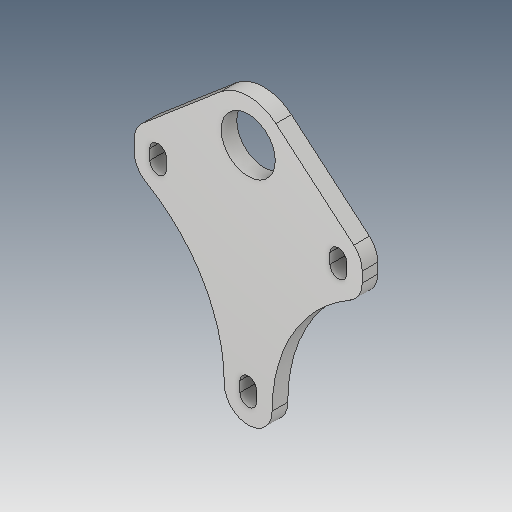
# Autodesk Inventor part: POTplate
Saved by Autodesk Inventor 2019.4 (Build 234330000, 330)
## iProperties
Created: 2019-06-16
Part Number: POTplate
Material: アルミニウム 2014-T4
Document SubType Name: Modeling
Designer: AzLIer
Density: 2.8 g/cm^3
Appearance: サテン
Mass: 11.1022 g
Surface Area: 33.0768 cm^2
Volume: 3.96506 cm^3
Author: AzLIer
Autodesk Inventor part; units mm, degrees
ref_plane "YZ Plane" through (0, 0, 0) normal (1, 0, 0) x (0, 1, 0)
ref_plane "XZ Plane" through (0, 0, 0) normal (0, 1, 0) x (-1, 0, 0)
ref_plane "XY Plane" through (0, 0, 0) normal (0, 0, 1) x (1, 0, 0)
sketch "スケッチ1" plane through (0, 0, 0) normal (0, 0, 1) x (1, 0, 0)
  circle A0 centre (0, 0) radius 5.2
  line L0 (25, -50) -> (-25, -50)
  line L1 (-25, -50) -> (-25, 50)
  line L2 (-25, 50) -> (25, 50)
  line L3 (25, 50) -> (25, -50)
  line L4 (25, -50) -> (-25, 50) construction
  line L5 (-25, -50) -> (25, 50) construction
  dimension "d0" = 10.4
  dimension "d1" = 50
  dimension "d2" = 100
  constraints: 12 end point, 2 midpoint, 2 parallel, 1 centre point, 1 coincident, 1 horizontal, 1 perpendicular
  measures "d0" diameter of A0
  measures "d1" distance of L1.end L2.end
  measures "d2" distance of L0.end L1.end
extrude "押し出し1" add sketch "スケッチ1" along normal blind 3
sketch "スケッチ2" plane through (0, 0, 3) normal (0, 0, 1) x (1, 0, 0)
  circle A0 centre (17.3198, -9.9987) radius 1.25 construction
  circle A1 centre (-17.3213, -10.0013) radius 1.25 construction
  circle A2 centre (0.0015, -40) radius 1.25 construction
  line L0 (-17.3213, -10.0013) -> (-17.3213, -12.0013) construction
  line L1 (-18.9213, -10.0013) -> (-18.9213, -12.0013)
  line L2 (-15.7213, -12.0013) -> (-15.7213, -10.0013)
  arc A3 (-15.7213, -10.0013) -> (-18.9213, -10.0013) centre (-17.3213, -10.0013) ccw
  arc A4 (-18.9213, -12.0013) -> (-15.7213, -12.0013) centre (-17.3213, -12.0013) ccw
  line L3 (0.0015, -40) -> (0.0015, -42) construction
  line L4 (-1.5985, -40) -> (-1.5985, -42)
  line L5 (1.6015, -42) -> (1.6015, -40)
  arc A5 (1.6015, -40) -> (-1.5985, -40) centre (0.0015, -40) ccw
  arc A6 (-1.5985, -42) -> (1.6015, -42) centre (0.0015, -42) ccw
  line L6 (17.3198, -9.9987) -> (17.3198, -11.9987) construction
  line L7 (15.7198, -9.9987) -> (15.7198, -11.9987)
  line L8 (18.9198, -11.9987) -> (18.9198, -9.9987)
  arc A7 (18.9198, -9.9987) -> (15.7198, -9.9987) centre (17.3198, -9.9987) ccw
  arc A8 (15.7198, -11.9987) -> (18.9198, -11.9987) centre (17.3198, -11.9987) ccw
  circle A9 centre (0, 0) radius 5.2 projected
  arc A10 (5.3111, 6.2476) -> (-5.3114, 6.2473) centre (0, 0) ccw
  line L9 (-12.7213, -12.0013) -> (-12.7213, -10.0013)
  arc A11 (-20.3008, -6.4967) -> (-21.9213, -10.0013) centre (-17.3213, -10.0013) ccw
  line L10 (-21.9213, -10.0013) -> (-21.9213, -12.0013)
  arc A12 (-21.9213, -12.0013) -> (-21.3048, -14.3016) centre (-17.3213, -12.0013) ccw
  line L11 (21.9198, -11.9987) -> (21.9198, -9.9987)
  arc A13 (21.9198, -9.9987) -> (20.2992, -6.494) centre (17.3198, -9.9987) ccw
  line L12 (12.7198, -9.9987) -> (12.7198, -11.9987)
  arc A14 (21.3037, -14.2984) -> (21.9198, -11.9987) centre (17.3198, -11.9987) ccw
  line L13 (4.6015, -40) -> (4.6015, -42)
  arc A15 (-3.9821, -44.3003) -> (3.9854, -44.2997) centre (0.0015, -42) ccw
  line L14 (-4.5985, -42) -> (-4.5985, -40)
  arc A16 (4.6015, -40) -> (-4.5985, -40) centre (0.0015, -40) ccw
  line L15 (-20.3008, -6.4967) -> (-5.3114, 6.2473)
  line L16 (5.3111, 6.2476) -> (20.2992, -6.494)
  line L17 (21.3037, -14.2984) -> (3.9854, -44.2997)
  line L18 (-3.9821, -44.3003) -> (-21.3048, -14.3016)
  point P0 (-17.3213, -11.0013)
  point P1 (0.0015, -41)
  point P2 (17.3198, -10.9987)
  dimension "d5" = 1.6
  dimension "d6" = 2
  dimension "d7" = 3
  dimension "d8" = 3
  dimension "d9" = 3
  dimension "d10" = 3
  constraints: 44 end point, 26 point on circle, 20 tangent, 13 centre point, 10 parallel, 3 midpoint, 2 equal radius, 1 vertical, 1 other
  measures "d5" radius of A4
  measures "d6" distance of L3.start L3.end
  measures "d7" radial gap between concentric circles of A9 A10
  measures "d8" radial gap between concentric circles of A4 A12
  measures "d9" radial gap between concentric circles of A8 A14
  measures "d10" distance between parallel lines of L5 L13
extrude "押し出し2" cut sketch "スケッチ2" against normal blind 3 keep common part
sketch "スケッチ3" plane through (0, 0, 3) normal (0, 0, 1) x (1, 0, 0)
  arc A0 (15.7198, -11.9987) -> (18.9198, -11.9987) centre (17.3198, -11.9987) ccw projected
  line L0 (15.7198, -9.9987) -> (15.7198, -11.9987) projected
  arc A1 (18.9198, -9.9987) -> (15.7198, -9.9987) centre (17.3198, -9.9987) ccw projected
  line L1 (18.9198, -11.9987) -> (18.9198, -9.9987) projected
  arc A2 (-1.5985, -42) -> (1.6015, -42) centre (0.0015, -42) ccw projected
  line L2 (-1.5985, -40) -> (-1.5985, -42) projected
  arc A3 (1.6015, -40) -> (-1.5985, -40) centre (0.0015, -40) ccw projected
  line L3 (1.6015, -42) -> (1.6015, -40) projected
  arc A4 (-18.9213, -12.0013) -> (-15.7213, -12.0013) centre (-17.3213, -12.0013) ccw projected
  line L4 (-18.9213, -10.0013) -> (-18.9213, -12.0013) projected
  arc A5 (-15.7213, -10.0013) -> (-18.9213, -10.0013) centre (-17.3213, -10.0013) ccw projected
  line L5 (-15.7213, -12.0013) -> (-15.7213, -10.0013) projected
  line L6 (-21.9213, -12.0013) -> (-21.9213, -10.0013) projected
  arc A6 (-21.9213, -12.0013) -> (-21.3048, -14.3016) centre (-17.3213, -12.0013) ccw projected
  line L7 (-3.9821, -44.3003) -> (-21.3048, -14.3016) projected
  arc A7 (-3.9821, -44.3003) -> (3.9854, -44.2997) centre (0.0015, -42) ccw projected
  line L8 (21.3037, -14.2984) -> (3.9854, -44.2997) projected
  arc A8 (21.3037, -14.2984) -> (21.9198, -11.9987) centre (17.3198, -11.9987) ccw projected
  line L9 (21.9198, -9.9987) -> (21.9198, -11.9987) projected
  arc A9 (21.9198, -9.9987) -> (20.2992, -6.494) centre (17.3198, -9.9987) ccw projected
  line L10 (5.3111, 6.2476) -> (20.2992, -6.494) projected
  arc A10 (5.3111, 6.2476) -> (-5.3114, 6.2473) centre (0, 0) ccw projected
  line L11 (-20.3008, -6.4967) -> (-5.3114, 6.2473) projected
  arc A11 (-20.3008, -6.4967) -> (-21.9213, -10.0013) centre (-17.3213, -10.0013) ccw projected
  circle A12 centre (0, 0) radius 5.2 projected
  arc A13 (19.6173, -15.9838) -> (4.6015, -41.9965) centre (34.6015, -41.9737) ccw
  arc A14 (19.6173, -15.9838) -> (21.3037, -14.2984) centre (17.3198, -11.9987) ccw
  arc A15 (-21.3048, -14.3016) -> (-19.6182, -15.9868) centre (-17.3213, -12.0013) ccw
  arc A16 (-4.5985, -41.9972) -> (-19.6182, -15.9868) centre (-34.5985, -41.9789) ccw
  arc A17 (-4.5985, -41.9972) -> (-3.9821, -44.3003) centre (0.0015, -42) ccw
  arc A18 (3.9854, -44.2997) -> (4.6015, -41.9965) centre (0.0015, -42) ccw
  arc A19 (-21.9213, -12.0013) -> (-21.3048, -14.3016) centre (-17.3213, -12.0013) ccw projected
  dimension "d14" = 30
  constraints: 12 point on circle, 6 centre point, 4 end point, 4 tangent, 3 coincident, 3 equal radius, 2 point on line
  measures "d14" radius of A13
extrude "押し出し3" cut sketch "スケッチ3" against normal through all contours L6 A11 L11 A10 L10 A9 L9 A8 A14 A13 A18 A7 A17 A16 A15 A6 keep common part
